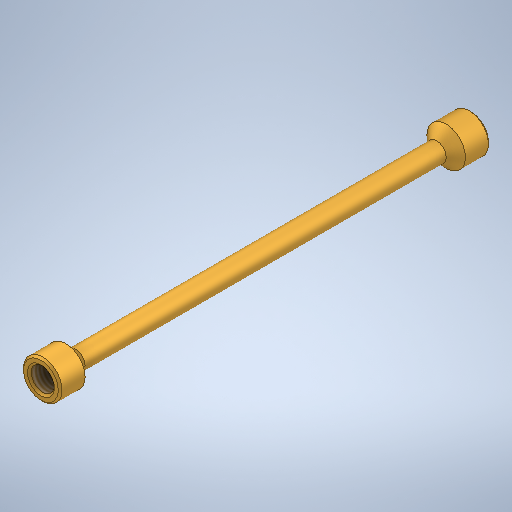
# Autodesk Inventor part: Heater
Saved by Autodesk Inventor 2025.2 (Build 292293000, 293)
## iProperties
Created: 2026-06-11
Part Number: Heater
Material: Generic
Document SubType Name: Modeling
Designer: Simon
Density: 1 g/cm^3
Appearance: Brass - Satin
Author: Simon
Autodesk Inventor part; units mm, degrees
ref_plane "YZ Plane" through (0, 0, 0) normal (1, 0, 0) x (0, 1, 0)
ref_plane "XZ Plane" through (0, 0, 0) normal (0, 1, 0) x (-1, 0, 0)
ref_plane "XY Plane" through (0, 0, 0) normal (0, 0, 1) x (1, 0, 0)
sketch "Sketch1" plane through (0, 0, 0) normal (1, 0, 0) x (0, 1, 0)
  line L0 (0, 0) -> (0, -112)
  line L1 (0, -112) -> (3, -112)
  line L2 (3, -112) -> (3, 0)
  line L3 (3, 0) -> (0, 0)
  line L4 (3, 0) -> (3, -6)
  line L5 (3, -112) -> (3, -106)
  line L6 (3, -112) -> (5, -112)
  line L7 (5, -112) -> (5, -106)
  line L8 (5, -106) -> (3, -106)
  line L9 (3, 0) -> (5, 0)
  line L10 (5, 0) -> (5, -6)
  line L11 (5, -6) -> (3, -6)
  line L12 (3, -106) -> (0.5, -106)
  line L13 (0.5, -106) -> (0.5, -6)
  line L14 (0.5, -6) -> (3, -6)
  line L15 (5, -6) -> (5, -7)
  line L16 (5, -7) -> (0.5, -7)
  line L17 (5, -106) -> (5, -105)
  line L18 (5, -105) -> (0.5, -105)
  line L19 (3, -7) -> (3.1, -7)
  line L20 (2.5, -7) -> (2.5, -105)
  point P0 (3, -105)
  point P1 (2, -6)
  point P2 (3.1, -105)
  dimension "d0" = 112
  dimension "d1" = 3
  dimension "d2" = 6
  dimension "d3" = 6
  dimension "d5" = 2
  dimension "d6" = 2
  dimension "d7" = 2.5
  dimension "d8" = 1
  dimension "d9" = 1
  dimension "d22" = 2
  constraints: 42 end point, 13 point on line, 10 perpendicular, 2 vertical, 1 horizontal, 1 parallel
  measures "d0" distance of L0.start L0.end
  measures "d1" distance of L0.end L1.end
  measures "d2" distance of L2.end L4.end
  measures "d3" distance of L1.end L5.end
  measures "d5" distance of L1.end L6.end
  measures "d6" distance of L2.end L9.end
  measures "d7" distance of L5.end L12.end
  measures "d8" distance of L10.end L15.end
  measures "d9" distance of L7.end L17.end
  measures "d22" distance between parallel lines of L20 L13
revolve "Revolution1" add sketch "Sketch1" angle 360 about axis through (0, 0, 0) along (0, 0, -1) contours L9 L10 L11 L2 | L2 L8 L7 L6 | L11 L15 L16 L2 | L2 L16 L13 L14 | L12 L13 L18 L2 | L2 L18 L17 L8 | L20 L18 L13 L16
thread "Thread1" size "M6x1" class "6H" standard "ANSI Metric M Profile" full length
thread "Thread2" size "M6x1" class "6H" standard "ANSI Metric M Profile" full length
chamfer "Chamfer1" distance 0.5 angle 45 2 edges at (0, -3, 0) (0, -3, -112)
chamfer "Chamfer2" distance 0.5 angle 45 4 edges at (0, -5, -112) (0, -5, -105) (0, -5, -7) (0, -5, 0)
chamfer "Chamfer3" distance 2 angle 45 2 edges at (0, -2.5, -7) (0, -2.5, -105)
body "Solid1"
